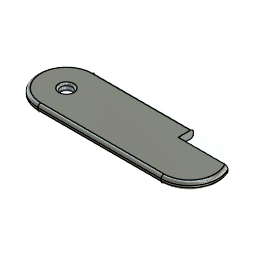
Bottle Cap opener (Autodesk Fusion 360 design; units mm, degrees)
part number: 2026-06-29-16-33-23-961
Autodesk Fusion 360 part; units mm, degrees
sketch "Sketch1" plane through (0, 0, 0) normal (0, 1, 0) x (1, 0, 0)
  line L0 (0, 0) -> (80, 0)
  line L1 (0, 0) -> (0, -65)
  line L2 (0, -65) -> (80, 0)
  dimension "d1" = 80
  dimension "d2" = 65
  constraint coincident L0.start L1.start
  constraint horizontal L0
  constraint perpendicular L0 L1
  measures "d1" distance of L0.start L0.end
  measures "d2" distance of L0.start L1.end
sketch "Sketch2" plane through (0, 0, 0) normal (0, 0, 1) x (1, 0, 0)
sketch "Sketch3" plane through (0, 0, 0) normal (0, 0, 1) x (1, 0, 0)
sketch "Sketch4" plane through (0, 0, 0) normal (0, 0, 1) x (1, 0, 0)
  line L0 (0, -15) -> (65, -15)
  arc A0 (65, -15) -> (65, 15) centre (65, 0) ccw
  line L1 (65, 15) -> (0, 15)
  arc A1 (0, 15) -> (0, -15) centre (0, 0) ccw
  line L2 (0, 0) -> (65, 0) construction
  dimension "d10" = 65
  dimension "d11" = 30
  constraint tangent L0 A0
  constraint tangent A0 L1
  constraint parallel L0 L1
  constraint tangent L1 A1
  constraint tangent L0 A1
  constraint horizontal L2
  constraint coincident A1.centre L2.start
  measures "d10" distance of A1.centre A0.centre
  measures "d11" diameter of A0
extrude "Extrude2" add sketch "Sketch4" along normal blind 4
sketch "Sketch5" plane through (0, 0, 4) normal (0, 0, 1) x (-1, 0, 0)
  arc A0 (0, -15) -> (0, 15) centre (0, 0) ccw
  line L0 (0, 15) -> (-65, 15)
  arc A1 (-65, 15) -> (-65, -15) centre (-65, 0) ccw
  line L1 (-65, -15) -> (0, -15)
sketch "Sketch6" plane through (0, 0, 4) normal (0, 0, 1) x (-1, 0, 0)
sketch "Sketch7" plane through (0, 0, 4) normal (0, 0, 1) x (-1, 0, 0)
  line L0 (-80, -15) -> (-52, -15)
  line L1 (-52, -15) -> (-52, -7)
  line L2 (-52, -7) -> (-80, -7)
  line L3 (-80, -7) -> (-80, -15)
  dimension "d18" = 28
  dimension "d19" = 8
  constraint horizontal L0
  constraint vertical L1
  constraint horizontal L2
  constraint vertical L3
  measures "d18" distance of L0.start L0.end
  measures "d19" distance of L0.start L2.end
extrude "Extrude3" cut sketch "Sketch7" against normal blind 4
sketch "Sketch8" plane through (0, 0, 4) normal (0, 0, 1) x (-1, 0, 0)
  circle A0 centre (0, 0) radius 3
  dimension "d22" = 6
  constraint coincident A0.centre origin
  measures "d22" diameter of A0
extrude "Extrude4" cut sketch "Sketch8" against normal blind 4
fillet "Fillet1" radius 1.5 8 edges at (26, 15, 4) (-15, 0, 4) (32.5, -15, 4) (77.8452, -7.746, 4) (26, 15, 0) (-15, 0, 0) (32.5, -15, 0) (77.8452, -7.746, 0)
fillet "Fillet2" radius 1 2 edges at (2.797, 1.0848, 0) (2.797, -1.0848, 4)
